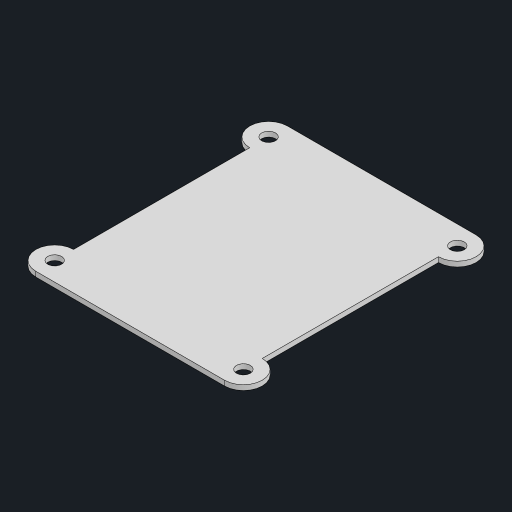
# Autodesk Inventor part: kiban
Saved by Autodesk Inventor 2023 (Build 270158000, 158)
## iProperties
Created: 2022-07-12
Part Number: kiban
Material: 一般
Document SubType Name: Modeling
Designer: legot
Density: 1 g/cm^3
Appearance: 既定
Author: legot
Autodesk Inventor part; units mm, degrees
ref_plane "YZ Plane" through (0, 0, 0) normal (1, 0, 0) x (0, 1, 0)
ref_plane "XZ Plane" through (0, 0, 0) normal (0, 1, 0) x (-1, 0, 0)
ref_plane "XY Plane" through (0, 0, 0) normal (0, 0, 1) x (1, 0, 0)
sketch "スケッチ1" plane through (0, 0, 0) normal (0, 1, 0) x (-1, 0, 0)
  line L0 (15, 20) -> (-15, 20)
  line L1 (-15, 20) -> (-15, -20)
  line L2 (-15, -20) -> (15, -20)
  line L3 (15, -20) -> (15, 14)
  arc A0 (15, 14) -> (15, 20) centre (15, 17) ccw
  line L4 (0, -20) -> (0, 20)
  line L5 (15, 0) -> (-15, 0)
  line L6 (15, 14) -> (15, 20) construction
  circle A1 centre (15, 17) radius 1.1
  arc A2 (15, 20) -> (15, 14) centre (15, 17) ccw construction
  point P0 (0, 0)
  point P1 (0, 0)
  dimension "d0" = 30
  dimension "d1" = 40
  dimension "d2" = 6
  dimension "d3" = 2.2
  constraints: 14 end point, 4 midpoint, 4 point on circle, 3 centre point, 3 parallel, 2 horizontal, 1 coincident, 1 horizontal alignment, 1 perpendicular, 1 point on line, 1 vertical, 1 vertical alignment
  measures "d0" distance of L0.start L0.end
  measures "d1" distance of L2.end L0.start
  measures "d2" diameter of A0
  measures "d3" diameter of A1
extrude "押し出し1" add sketch "スケッチ1" along normal blind 0.8 contours A0 L3 L5 L4 L0
mirror "ミラー1" about plane through (0, 0, 20) normal (1, 0, 0) of "押し出し1"
mirror "ミラー2" about plane through (0, 0, 0) normal (0, 0, -1) of "押し出し1", "ミラー1"
